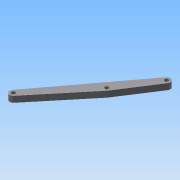
# Autodesk Inventor part: 1-3
Saved by Autodesk Inventor 2015 (Build 190159000, 159)
## iProperties
Created: 2018-05-07
Part Number: 1-3
Material: 一般
Document SubType Name: Modeling
Designer: 王博聖
Density: 1 g/cm^3
Appearance: 預設
Author: 王博聖
Autodesk Inventor part; units mm, degrees
ref_plane "YZ Plane" through (0, 0, 0) normal (1, 0, 0) x (0, 1, 0)
ref_plane "XZ Plane" through (0, 0, 0) normal (0, 1, 0) x (-1, 0, 0)
ref_plane "XY Plane" through (0, 0, 0) normal (0, 0, 1) x (1, 0, 0)
sketch "草圖1" plane through (0, 0, 0) normal (0, 0, 1) x (1, 0, 0)
  line L0 (0, 0) -> (14.1158, 17.1084)
  line L1 (14.1158, 17.1084) -> (21.9637, 29.2772)
  line L2 (21.9637, 29.2772) -> (0, 0)
  line L3 (14.1158, 17.1084) -> (0, 0) construction
  line L4 (13.1516, 17.9039) -> (-0.9642, 0.7955)
  line L5 (0.9642, -0.7955) -> (15.08, 16.3128)
  arc A0 (15.08, 16.3128) -> (13.1516, 17.9039) centre (14.1158, 17.1084) ccw
  arc A1 (-0.9642, 0.7955) -> (0.9642, -0.7955) centre (0, 0) ccw
  line L6 (21.9637, 29.2772) -> (14.1158, 17.1084) construction
  line L7 (20.9132, 29.9547) -> (13.0653, 17.7859)
  line L8 (15.1663, 16.4309) -> (23.0142, 28.5998)
  arc A2 (23.0142, 28.5998) -> (20.9132, 29.9547) centre (21.9637, 29.2772) ccw
  arc A3 (13.0653, 17.7859) -> (15.1663, 16.4309) centre (14.1158, 17.1084) ccw
  line L9 (21.9637, 29.2772) -> (0, 0) construction
  line L10 (20.9638, 30.0274) -> (-0.9999, 0.7501)
  line L11 (0.9999, -0.7501) -> (22.9636, 28.5271)
  arc A4 (22.9636, 28.5271) -> (20.9638, 30.0274) centre (21.9637, 29.2772) ccw
  arc A5 (-0.9999, 0.7501) -> (0.9999, -0.7501) centre (0, 0) ccw
  point P0 (7.0579, 8.5542)
  point P1 (18.0397, 23.1928)
  point P2 (10.9818, 14.6386)
  dimension "d0" = 22.18
  dimension "d1" = 14.48
  dimension "d2" = 36.6
  dimension "d3" = 2.5
  dimension "d4" = 2.5
  dimension "d5" = 2.5
  constraints: 30 end point, 12 point on circle, 12 tangent, 6 centre point, 5 equal length, 3 midpoint, 2 concentric
  measures "d0" distance of L0.start L0.end
  measures "d1" distance of L0.end L1.end
  measures "d2" distance of L0.start L1.end
  measures "d3" diameter of A1
  measures "d4" diameter of A3
  measures "d5" diameter of A5
extrude "擠出1" add sketch "草圖1" along normal blind 2
sketch "草圖2" plane through (0, 0, 2) normal (0, 0, 1) x (1, 0, 0)
  arc A0 (15.08, 16.3128) -> (15.1663, 16.4309) centre (14.1158, 17.1084) ccw projected
  arc A1 (23.0142, 28.5998) -> (20.9638, 30.0274) centre (21.9637, 29.2772) ccw projected
  arc A2 (-0.9999, 0.7501) -> (0.9642, -0.7955) centre (0, 0) ccw projected
  circle A3 centre (14.1158, 17.1084) radius 0.625
  circle A4 centre (21.9637, 29.2772) radius 0.625
  circle A5 centre (0, 0) radius 0.625
  dimension "d8" = 1.25
  dimension "d9" = 1.25
  dimension "d10" = 1.25
  constraints: 3 centre point, 3 coincident
  measures "d8" diameter of A3
  measures "d9" diameter of A4
  measures "d10" diameter of A5
extrude "擠出2" cut sketch "草圖2" against normal blind 2
